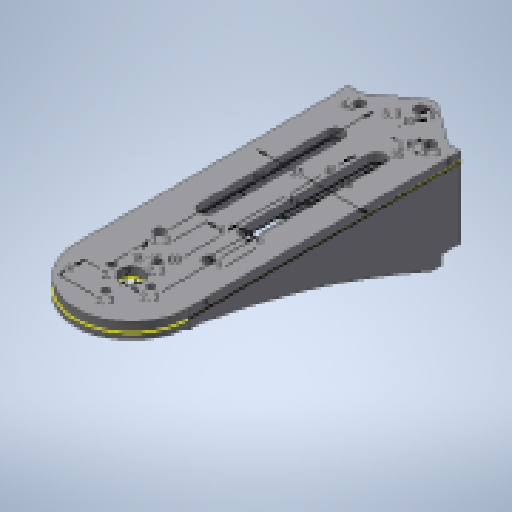
# Autodesk Inventor part: 机臂
Saved by Autodesk Inventor 2025.2 (Build 292293000, 293)
## iProperties
Created: 2026-03-18
Part Number: 机臂
Material: 常规
Document SubType Name: Modeling
Designer: BO‘S_SLAVE
Density: 1 g/cm^3
Appearance: 默认
Author: BO‘S_SLAVE
Autodesk Inventor part; units mm, degrees
ref_plane "YZ Plane" through (0, 0, 0) normal (1, 0, 0) x (0, 1, 0)
ref_plane "XZ Plane" through (0, 0, 0) normal (0, 1, 0) x (-1, 0, 0)
ref_plane "XY Plane" through (0, 0, 0) normal (0, 0, 1) x (1, 0, 0)
sketch "草图1" plane through (0, 0, 0) normal (0, 1, 0) x (-1, 0, 0)
  line L0 (17.5, -42.5) -> (-17.5, -42.5)
  line L1 (-17.5, -42.5) -> (-17.5, 42.5)
  line L2 (-17.5, 42.5) -> (17.5, 42.5)
  line L3 (17.5, 42.5) -> (17.5, -42.5)
  line L4 (0, 42.5) -> (0, -42.5)
  line L5 (17.5, 0) -> (-17.5, 0)
  arc A0 (17.5, 42.5) -> (-17.5, 42.5) centre (0, 42.5) ccw
  circle A1 centre (0, 42.5) radius 3.5
  circle A2 centre (0, 34.5) radius 1.15
  circle A3 centre (0, 50.5) radius 1.15
  circle A4 centre (8, 42.5) radius 1.15
  circle A5 centre (-8, 42.5) radius 1.15
  line L6 (0, 50.5) -> (0, 34.5)
  line L7 (-8, 42.5) -> (8, 42.5)
  circle A6 centre (7.6071, 26.1865) radius 1.65
  line L8 (7.6071, 26.1865) -> (0, 42.5)
  circle A7 centre (-7.6071, 26.1865) radius 1.65
  line L9 (-7.6071, 26.1865) -> (0, 42.5)
  line L10 (13.5, -42.5) -> (0, -52.5)
  line L11 (0, -52.5) -> (-13.5, -42.5)
  line L12 (0, 7.5) -> (0, -22.5) construction
  line L13 (-6.5, 12.5) -> (-6.5, -27.5) construction
  line L14 (-9, 12.5) -> (-9, -27.5)
  line L15 (-4, -27.5) -> (-4, 12.5)
  arc A8 (-4, 12.5) -> (-9, 12.5) centre (-6.5, 12.5) ccw
  arc A9 (-9, -27.5) -> (-4, -27.5) centre (-6.5, -27.5) ccw
  line L16 (9, 12.5) -> (9, -27.5)
  line L17 (4, -27.5) -> (4, 12.5)
  arc A10 (9, 12.5) -> (4, 12.5) centre (6.5, 12.5) ccw
  arc A11 (4, -27.5) -> (9, -27.5) centre (6.5, -27.5) ccw
  circle A12 centre (-11, -39.5) radius 1.65
  line L18 (0, 12.5) -> (0, -27.5) construction
  line L19 (0, -7.5) -> (-6.5, -7.5)
  line L20 (0, -42.5) -> (0, -52.5)
  circle A13 centre (0, -47.5) radius 1.65
  circle A14 centre (11, -39.5) radius 1.65
  line L21 (0, 34.5) -> (8, 42.5)
  line L22 (0, 50.5) -> (8, 42.5)
  line L23 (0, 50.5) -> (-8, 42.5)
  line L24 (-8, 42.5) -> (0, 34.5)
  point P0 (0, 0)
  point P1 (0, 0)
  dimension "d0" = 7
  dimension "d1" = 2.3
  dimension "d2" = 2.3
  dimension "d3" = 2.3
  dimension "d4" = 2.3
  dimension "d5" = 8
  dimension "d6" = 8
  dimension "d7" = 8
  dimension "d8" = 35
  dimension "d9" = 85
  dimension "d13" = 3.3
  dimension "d14" = 18
  dimension "d15" = 25
  dimension "d29" = 40
  dimension "d30" = 5
  dimension "d31" = 35
  dimension "d33" = 10
  dimension "d34" = 4
  dimension "d43" = 3.3
  dimension "d48" = 40
  dimension "d58" = 3.3
  dimension "d59" = 5
  dimension "d65" = 11
  dimension "d66" = 3
  dimension "d67" = 4
  dimension "d68" = 4
  constraints: 56 end point, 15 centre point, 12 midpoint, 10 point on circle, 8 symmetric about line, 7 coincident, 5 parallel, 4 point on line, 4 tangent, 2 horizontal, 2 vertical, 1 collinear, 1 equal length, 1 perpendicular, 4 other
  measures "d0" diameter of A1
  measures "d1" diameter of A2
  measures "d2" diameter of A3
  measures "d3" diameter of A4
  measures "d4" diameter of A5
  measures "d5" distance of A1.centre A3.centre
  measures "d6" distance from line of L6 A4.centre
  measures "d7" distance from line of L6 A5.centre
  measures "d8" distance between parallel lines of L1 L3
  measures "d9" distance between parallel lines of L2 L0
  measures "d13" diameter of A6
  measures "d14" distance of L8.start L8.end
  measures "d15" angle of L4 L8
  measures "d29" distance of L13.start L13.end
  measures "d30" distance between parallel lines of L15 L14
  measures "d31" distance from line of L0 L19.end
  measures "d33" distance from line of L0 L10.end
  measures "d34" distance between parallel lines of L4 L15
  measures "d43" diameter of A12
  measures "d48" distance of L18.start L18.end
  measures "d58" diameter of A13
  measures "d59" distance of L10.end A13.centre
  measures "d65" distance from line of L4 A12.centre
  measures "d66" distance from line of A12.centre L0
  measures "d67" distance of L0.start L10.start
  measures "d68" distance of L0.end L11.end
extrude "拉伸1" add sketch "草图1" along normal blind 3 contours L0 L4 L5 L17 A11 L16 L3 | L10 L20 A13 L0 | L5 L16 A10 L17 L4 A2 L21 A4 L2 L3 | L20 A13 L11 L0 | L0 L1 L5 L14 A9 L15 L19 L4 | L2 A4 L22 A3 L23 A5 A0 | L19 L15 L5 L4 | L2 A5 L24 A2 L4 L5 L15 A8 L14 L1 | A4 L2 A1 L6 A3 L22 | L21 L8 A1 L2 A4 | L21 A2 L4 A1 L8 | L23 A3 L6 A1 L2 A5 | A5 L2 A1 L9 L24 | L24 L9 A1 L4 A2
sketch "草图2" plane through (0, 0, 0) normal (0, -1, 0) x (1, 0, 0)
  circle A0 centre (0, 42.5) radius 3.5 projected
  arc A1 (17.5, 42.5) -> (-17.5, 42.5) centre (0, 42.5) ccw projected
  line L0 (13.5, 42.5) -> (-13.5, 42.5)
  arc A2 (13.5, 42.5) -> (-13.5, 42.5) centre (0, 42.5) ccw
  line L1 (13.5, 42.5) -> (17.5, 42.5)
  line L2 (-13.5, 42.5) -> (-17.5, 42.5)
  line L3 (13.5, 42.5) -> (13.5, -42.5)
  line L4 (-13.5, -42.5) -> (-13.5, 42.5)
  line L5 (17.5, 42.5) -> (17.5, -42.5) projected
  line L6 (-17.5, -42.5) -> (-17.5, 42.5) projected
  line L7 (-13.5, -42.5) -> (-17.5, -42.5) projected
  line L8 (17.5, -42.5) -> (13.5, -42.5) projected
  line L9 (13.5, -42.5) -> (-13.5, -42.5)
  line L10 (13.5, -36.5) -> (-13.5, -36.5)
  circle A3 centre (11, -39.5) radius 1.65 projected
  circle A4 centre (-11, -39.5) radius 1.65 projected
  point P0 (0, 0)
  dimension "d69" = 4
  dimension "d70" = 6
  constraints: 14 end point, 4 equal length, 4 point on line, 3 horizontal, 2 midpoint, 2 perpendicular, 2 point on circle, 1 centre point, 1 coincident, 1 vertical
  measures "d69" distance between parallel lines of L5 L3
  measures "d70" distance between parallel lines of L9 L10
extrude "拉伸2" add sketch "草图2" along normal blind 2 contours A2 L2 A1 L1
extrude "拉伸3" add sketch "草图2" along normal blind 25 contours L1 L5 L8 L3 | L4 L7 L6 L2 | L3 L9 L4 L10
sketch "草图3" plane through (17.5, 3, 42.5) normal (1, 0, 0) x (0, 0, -1)
  line L0 (85, -28) -> (85, 0) projected
  line L1 (0, 0) -> (85, 0) projected
  line L2 (0, -5) -> (0, -28) projected
  line L3 (85, -28) -> (0, -28) projected
  line L4 (4, -4) -> (85, -4)
  line L5 (4, -4) -> (4, -6)
  line L6 (0, 0) -> (85, 0) projected
  line L7 (4, -6) -> (0, -6)
  line L8 (76, -4) -> (76, -28)
  arc A0 (76, -28) -> (4, -6) centre (-46.9727, -301.6379) ccw
  line L9 (0, -5) -> (0, 0) projected
  line L10 (79, -3) -> (79, -28) projected
  line L11 (79, -3) -> (79, 0)
  point P0 (42.5, -3)
  dimension "d50" = 4
  dimension "d51" = 4
  dimension "d52" = 6
  dimension "d53" = 9
  dimension "d57" = 300
  constraints: 10 end point, 5 point on line, 4 perpendicular, 2 point on circle, 1 centre point, 1 parallel, 1 vertical
  measures "d50" distance between parallel lines of L2 L5
  measures "d51" distance between parallel lines of L1 L4
  measures "d52" distance between parallel lines of L1 L7
  measures "d53" distance between parallel lines of L0 L8
  measures "d57" radius of A0
extrude "拉伸5" cut sketch "草图3" against normal blind 100 contours L3 L2 L7 A0
sketch "草图6" plane through (0, -25, 0) normal (0, -1, 0) x (1, 0, 0)
  line L0 (-13.5, -33.5) -> (-17.5, -33.5) projected
  line L1 (-17.5, -33.5) -> (-17.5, -42.5) projected
  line L2 (-17.5, -42.5) -> (17.5, -42.5) projected
  line L3 (17.5, -42.5) -> (17.5, -33.5) projected
  line L4 (17.5, -33.5) -> (13.5, -33.5) projected
  line L5 (13.5, -33.5) -> (13.5, -36.5) projected
  line L6 (13.5, -36.5) -> (-13.5, -36.5) projected
  line L7 (-13.5, -36.5) -> (-13.5, -33.5) projected
  circle A0 centre (-11, -39.5) radius 1.65 projected
  circle A1 centre (11, -39.5) radius 1.65 projected
  line L8 (13.5, -36.5) -> (17.5, -36.5)
  line L9 (17.5, -42.5) -> (17.5, -33.5) projected
  line L10 (-13.5, -36.5) -> (-17.5, -36.5)
  point P0 (0, 0)
  constraints: 4 end point, 3 point on line, 1 perpendicular
extrude "拉伸7" cut sketch "草图6" against normal blind 3 contours L6 L8 L3 L2 L1 L10
fillet "圆角1" radius 3 3 edges at (-13.5, 1.5, -42.5) (0, 1.5, -52.5) (13.5, 1.5, -42.5)
fillet "圆角2" radius 2 4 edges at (15.5, -2, 42.5) (15.5, -3, 42.5) (-15.5, -2, 42.5) (-15.5, -3, 42.5)
fillet "圆角3" radius 3 2 edges at (15.5, -25, -33.5) (-15.5, -25, -33.5)
sketch "草图7" plane through (17.5, -22, -42.5) normal (0, 0, -1) x (-1, 0, 0)
  line L0 (3.0099, 25) -> (3.0099, 22) projected
  line L1 (0, 25) -> (3.0099, 25) projected
  line L2 (0, 0) -> (0, 25) projected
  line L3 (0, 0) -> (35, 0) projected
  line L4 (35, 0) -> (35, 25) projected
  line L5 (31.9901, 25) -> (35, 25) projected
  line L6 (31.9901, 22) -> (31.9901, 25) projected
  line L7 (3.0099, 22) -> (31.9901, 22) projected
  line L8 (13.5, 6) -> (21.5, 6) construction
  line L9 (13.5, 9) -> (21.5, 9)
  line L10 (21.5, 3) -> (13.5, 3)
  arc A0 (13.5, 9) -> (13.5, 3) centre (13.5, 6) ccw
  arc A1 (21.5, 3) -> (21.5, 9) centre (21.5, 6) ccw
  point P0 (17.5, 22)
  point P1 (17.5, 6)
  dimension "d76" = 8
  dimension "d77" = 6
  dimension "d78" = 6
  dimension "d79" = 17.5
  constraints: 8 end point, 4 point on circle, 4 tangent, 2 centre point, 1 horizontal, 1 midpoint, 1 parallel
  measures "d76" distance of L8.start L8.end
  measures "d77" distance between parallel lines of L10 L9
  measures "d78" distance from line of L3 point (17.5, 6)
  measures "d79" distance from line of L4 point (17.5, 6)
extrude "拉伸8" cut sketch "草图7" against normal up to surface (6 mm away) contours L9 A1 L10 A0
fillet "圆角4" radius 2 4 edges at (0, 0, 56) (-13.5, 0, 3) (13.5, 0, 3) (0, 0, -36.5)
sketch "草图5" plane through (0, -12, 0) normal (0, -1, 0) x (1, 0, 0)
  line L0 (-13.5, -42.5) -> (13.5, -42.5) projected
  line L1 (-13.5, -42.5) -> (0, -62.5) projected
  line L2 (0, -62.5) -> (13.5, -42.5) projected
  circle A0 centre (0, -55.5) radius 1.65 projected
  circle A1 centre (6.5, -46.5) radius 1.65 projected
  line L3 (7.425, -51.5) -> (-7.425, -51.5)
  point P0 (0, 0)
  dimension "d60" = 11
  constraints: 2 end point, 2 point on line, 1 horizontal
  measures "d60" distance from line of L1.end L3
